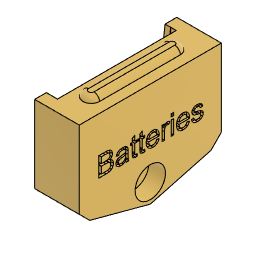
Battery_Cap (Autodesk Fusion 360 design; units mm, degrees)
Autodesk Fusion 360 part; units mm, degrees
(part 1 of 2)
sketch "Cap Face" plane through (-62, 0, 0) normal (-1, 0, 0) x (0, -1, 0)
  line L0 (0, -13.8691) -> (1.875, -15.7441)
  line L1 (1.875, -15.7441) -> (12.75, -18.6581)
  line L2 (12.75, -18.6581) -> (23.625, -15.7441)
  line L3 (23.625, -15.7441) -> (25.5, -13.8691)
  line L4 (0, 0) -> (25.5, 0)
  line L5 (25.5, 0) -> (25.5, -13.8691)
  line L6 (0, -13.8691) -> (0, 0)
  line L7 (0, -13.8691) -> (1.875, -15.7441)
  line L8 (1.875, -15.7441) -> (12.75, -18.6581)
  line L9 (12.75, -18.6581) -> (23.625, -15.7441)
  line L10 (23.625, -15.7441) -> (25.5, -13.8691)
  dimension "d72" = 13.8691
  dimension "d73" = 18.6581
  dimension "d74" = 25.5
  dimension "d75" = 10.875
  dimension "d76" = 10.875
  dimension "d77" = 1.875
  dimension "d78" = 1.875
  dimension "d79" = 1.875
  dimension "d80" = 1.875
  dimension "d81" = 2.9139
  dimension "d82" = 2.9139
  dimension "d83" = 150
  dimension "d84" = 150
  dimension "d85" = 135
  constraint coincident L4.start L6.end
  constraint horizontal L4
  constraint vertical L5
  constraint vertical L6
  constraint coincident L4.start L6
  constraint coincident L6.end L4
  constraint coincident L2 L1.end
  measures "d72" distance of L4.start L0.start
  measures "d73" vertical distance of L4.start L1.end
  measures "d74" distance of L4.start L4.end
  measures "d75" horizontal distance of L1.end L2.end
  measures "d76" horizontal distance of L0.end L1.end
  measures "d77" horizontal distance of L2.end L3.end
  measures "d78" horizontal distance of L0.end L0.start
  measures "d79" vertical distance of L2.end L3.end
  measures "d80" vertical distance of L0.end L0.start
  measures "d81" vertical distance of L1.end L2.end
  measures "d82" vertical distance of L0.end L1.end
  measures "d83" angle of L7 L8
  measures "d84" angle of L9 L10
  measures "d85" angle of L3 L5
extrude "Cap Extrusion" add sketch "Cap Face" along normal blind 8
sketch "Battery Label" plane through (-62, 0, 0) normal (1, 0, 0) x (0, 1, 0)
  line L0 (0, -13.8691) -> (0, 0)
  line L1 (0, 0) -> (-25.5, 0)
  line L2 (-25.5, 0) -> (-25.5, -13.8691)
  line L3 (-22, -10.5) -> (-3, -10.5) construction
  line L4 (-3, -10.5) -> (-3, -6.5) construction
  line L5 (-3, -6.5) -> (-22, -6.5) construction
  line L6 (-22, -6.5) -> (-22, -10.5) construction
  line L7 (-1.875, -15.7441) -> (0, -13.8691)
  line L8 (-25.5, -13.8691) -> (-23.625, -15.7441)
  line L9 (-23.625, -15.7441) -> (-12.75, -18.6581)
  line L10 (-12.75, -18.6581) -> (-1.875, -15.7441)
  dimension "d19" = 3.5
  dimension "d87" = 6.5
  dimension "d88" = 3.5
  dimension "d89" = 19
  dimension "d90" = 4
  text T0 "Batteries" font "Arial" height 3.5 align left top in box 19 x 4 at (-22, -10.5) x (1, 0) y (0, 1) spacing 1 kerned
  constraint parallel L1 L5
  measures "d87" distance of L1 L5
  measures "d88" distance of L2 L6
extrude "Label Cutout" cut sketch "Battery Label" against normal blind 0.5 text T0
sketch "Screw Hole" plane through (-62, 0, 0) normal (1, 0, 0) x (0, 1, 0)
  line L0 (0, -13.8691) -> (0, 0)
  line L1 (0, 0) -> (-25.5, 0)
  line L2 (-25.5, 0) -> (-25.5, -13.8691)
  spline S0 degree 3 poles (-20.1008, -9.9415) (-20.186, -9.9585) (-20.3723, -9.9958) (-20.5623, -9.9985) (-20.6654, -10) knots 0 0 0 0 0.026008 0.05687 0.05687 0.05687 0.05687
  line L3 (-20.6654, -10) -> (-22, -10)
  line L4 (-22, -10) -> (-22, -6.5)
  line L5 (-22, -6.5) -> (-20.6869, -6.5)
  spline S1 degree 3 poles (-20.6869, -6.5) (-20.5653, -6.5022) (-20.3453, -6.5062) (-20.1367, -6.5753) (-20.0435, -6.6062) knots 0 0 0 0 0.036237 0.065543 0.065543 0.065543 0.065543
  spline S2 degree 3 poles (-20.0435, -6.6062) (-19.9672, -6.6463) (-19.8153, -6.7259) (-19.7142, -6.8644) (-19.6639, -6.9333) knots 0 0 0 0 0.025471 0.050707 0.050707 0.050707 0.050707
  spline S3 degree 3 poles (-19.6639, -6.9333) (-19.6238, -7.0069) (-19.5453, -7.1513) (-19.5328, -7.3151) (-19.5266, -7.3953) knots 0 0 0 0 0.024827 0.048681 0.048681 0.048681 0.048681
  spline S4 degree 3 poles (-19.5266, -7.3953) (-19.5319, -7.4693) (-19.5425, -7.6188) (-19.6129, -7.7511) (-19.6484, -7.8179) knots 0 0 0 0 0.021997 0.044414 0.044414 0.044414 0.044414
  spline S5 degree 3 poles (-19.6484, -7.8179) (-19.6958, -7.8815) (-19.795, -8.0147) (-19.9402, -8.0956) (-20.016, -8.1378) knots 0 0 0 0 0.023539 0.049232 0.049232 0.049232 0.049232
  spline S6 degree 3 poles (-20.016, -8.1378) (-19.9177, -8.1726) (-19.7291, -8.2392) (-19.5929, -8.3854) (-19.5278, -8.4553) knots 0 0 0 0 0.030777 0.059013 0.059013 0.059013 0.059013
  spline S7 degree 3 poles (-19.5278, -8.4553) (-19.478, -8.5346) (-19.3762, -8.6966) (-19.3636, -8.8877) (-19.3571, -8.9853) knots 0 0 0 0 0.027618 0.056465 0.056465 0.056465 0.056465
  spline S8 degree 3 poles (-19.3571, -8.9853) (-19.3612, -9.0655) (-19.3694, -9.2239) (-19.4307, -9.3702) (-19.4609, -9.4425) knots 0 0 0 0 0.023867 0.0472 0.0472 0.0472 0.0472
  spline S9 degree 3 poles (-19.4609, -9.4425) (-19.4961, -9.5078) (-19.5627, -9.6315) (-19.6679, -9.7245) (-19.7176, -9.7684) knots 0 0 0 0 0.02202 0.041772 0.041772 0.041772 0.041772
  spline S10 degree 3 poles (-19.7176, -9.7684) (-19.7737, -9.8048) (-19.8926, -9.8817) (-20.0288, -9.9209) (-20.1008, -9.9415) knots 0 0 0 0 0.019941 0.042252 0.042252 0.042252 0.042252
  spline S11 degree 3 poles (-15.4524, -9.6013) (-15.4319, -9.6103) (-15.3853, -9.6308) (-15.3342, -9.6318) (-15.3056, -9.6323) knots 0 0 0 0 0.006657 0.015139 0.015139 0.015139 0.015139
  spline S12 degree 3 poles (-15.3056, -9.6323) (-15.2779, -9.6314) (-15.2148, -9.6291) (-15.1521, -9.6205) (-15.117, -9.6156) knots 0 0 0 0 0.008307 0.018945 0.018945 0.018945 0.018945
  line L6 (-15.117, -9.6156) -> (-15.0549, -9.9952)
  spline S13 degree 3 poles (-15.0549, -9.9952) (-15.112, -10.0064) (-15.2193, -10.0273) (-15.3285, -10.0315) (-15.3796, -10.0334) knots 0 0 0 0 0.017427 0.032736 0.032736 0.032736 0.032736
  spline S14 degree 3 poles (-15.3796, -10.0334) (-15.4499, -10.0321) (-15.5757, -10.0297) (-15.6914, -9.9809) (-15.7425, -9.9594) knots 0 0 0 0 0.020853 0.037334 0.037334 0.037334 0.037334
  spline S15 degree 3 poles (-15.7425, -9.9594) (-15.782, -9.9335) (-15.8584, -9.8834) (-15.9026, -9.8035) (-15.9239, -9.7648) knots 0 0 0 0 0.013927 0.026964 0.026964 0.026964 0.026964
  spline S16 degree 3 poles (-15.9239, -9.7648) (-15.939, -9.7027) (-15.9794, -9.5365) (-15.9776, -9.3649) (-15.9765, -9.2575) knots 0 0 0 0 0.019122 0.05117 0.05117 0.05117 0.05117
  line L7 (-15.9765, -9.2575) -> (-15.9765, -7.7988)
  line L8 (-15.9765, -7.7988) -> (-16.2916, -7.7988)
  line L9 (-16.2916, -7.7988) -> (-16.2916, -7.4645)
  line L10 (-16.2916, -7.4645) -> (-15.9765, -7.4645)
  line L11 (-15.9765, -7.4645) -> (-15.9765, -6.8366)
  line L12 (-15.9765, -6.8366) -> (-15.5491, -6.5788)
  line L13 (-15.5491, -6.5788) -> (-15.5491, -7.4645)
  line L14 (-15.5491, -7.4645) -> (-15.117, -7.4645)
  line L15 (-15.117, -7.4645) -> (-15.117, -7.7988)
  line L16 (-15.117, -7.7988) -> (-15.5491, -7.7988)
  line L17 (-15.5491, -7.7988) -> (-15.5491, -9.2814)
  spline S17 degree 3 poles (-15.5491, -9.2814) (-15.5497, -9.332) (-15.5507, -9.4118) (-15.5329, -9.4894) (-15.5264, -9.5177) knots 0 0 0 0 0.015111 0.023814 0.023814 0.023814 0.023814
  spline S18 degree 3 poles (-15.5264, -9.5177) (-15.5176, -9.5344) (-15.4996, -9.5682) (-15.4683, -9.5902) (-15.4524, -9.6013) knots 0 0 0 0 0.00558 0.011304 0.011304 0.011304 0.011304
  spline S19 degree 3 poles (-11.5477, -9.8424) (-11.6529, -9.905) (-11.876, -10.038) (-12.136, -10.0506) (-12.2735, -10.0573) knots 0 0 0 0 0.036142 0.076727 0.076727 0.076727 0.076727
  spline S20 degree 3 poles (-12.2735, -10.0573) (-12.4466, -10.0458) (-12.7775, -10.0239) (-13.0336, -9.8146) (-13.1557, -9.7147) knots 0 0 0 0 0.050598 0.096759 0.096759 0.096759 0.096759
  spline S21 degree 3 poles (-13.1557, -9.7147) (-13.2506, -9.5823) (-13.4557, -9.2963) (-13.4725, -8.9433) (-13.4816, -8.7538) knots 0 0 0 0 0.047865 0.103406 0.103406 0.103406 0.103406
  spline S22 degree 3 poles (-13.4816, -8.7538) (-13.4726, -8.5579) (-13.4561, -8.1943) (-13.2481, -7.8975) (-13.1521, -7.7606) knots 0 0 0 0 0.057415 0.106574 0.106574 0.106574 0.106574
  spline S23 degree 3 poles (-13.1521, -7.7606) (-13.0321, -7.6575) (-12.7864, -7.4464) (-12.463, -7.4205) (-12.2974, -7.4072) knots 0 0 0 0 0.046198 0.09464 0.09464 0.09464 0.09464
  spline S24 degree 3 poles (-12.2974, -7.4072) (-12.1368, -7.4204) (-11.8221, -7.4463) (-11.5834, -7.6525) (-11.4666, -7.7534) knots 0 0 0 0 0.047001 0.092108 0.092108 0.092108 0.092108
  spline S25 degree 3 poles (-14.094, -9.6013) (-14.0735, -9.6103) (-14.0268, -9.6308) (-13.9758, -9.6318) (-13.9471, -9.6323) knots 0 0 0 0 0.006657 0.015139 0.015139 0.015139 0.015139
  spline S26 degree 3 poles (-13.9471, -9.6323) (-13.9194, -9.6314) (-13.8563, -9.6291) (-13.7937, -9.6205) (-13.7585, -9.6156) knots 0 0 0 0 0.008307 0.018945 0.018945 0.018945 0.018945
  line L18 (-13.7585, -9.6156) -> (-13.6965, -9.9952)
  spline S27 degree 3 poles (-13.6965, -9.9952) (-13.7536, -10.0064) (-13.8609, -10.0273) (-13.9701, -10.0315) (-14.0211, -10.0334) knots 0 0 0 0 0.017427 0.032736 0.032736 0.032736 0.032736
  spline S28 degree 3 poles (-14.0211, -10.0334) (-14.0914, -10.0321) (-14.2173, -10.0297) (-14.333, -9.9809) (-14.384, -9.9594) knots 0 0 0 0 0.020853 0.037334 0.037334 0.037334 0.037334
  spline S29 degree 3 poles (-14.384, -9.9594) (-14.4235, -9.9335) (-14.4999, -9.8834) (-14.5441, -9.8035) (-14.5655, -9.7648) knots 0 0 0 0 0.013927 0.026964 0.026964 0.026964 0.026964
  spline S30 degree 3 poles (-14.5655, -9.7648) (-14.5806, -9.7027) (-14.621, -9.5365) (-14.6192, -9.3649) (-14.618, -9.2575) knots 0 0 0 0 0.019122 0.05117 0.05117 0.05117 0.05117
  line L19 (-14.618, -9.2575) -> (-14.618, -7.7988)
  line L20 (-14.618, -7.7988) -> (-14.9332, -7.7988)
  line L21 (-14.9332, -7.7988) -> (-14.9332, -7.4645)
  line L22 (-14.9332, -7.4645) -> (-14.618, -7.4645)
  line L23 (-14.618, -7.4645) -> (-14.618, -6.8366)
  line L24 (-14.618, -6.8366) -> (-14.1907, -6.5788)
  line L25 (-14.1907, -6.5788) -> (-14.1907, -7.4645)
  line L26 (-14.1907, -7.4645) -> (-13.7585, -7.4645)
  line L27 (-13.7585, -7.4645) -> (-13.7585, -7.7988)
  line L28 (-13.7585, -7.7988) -> (-14.1907, -7.7988)
  line L29 (-14.1907, -7.7988) -> (-14.1907, -9.2814)
  spline S31 degree 3 poles (-14.1907, -9.2814) (-14.1913, -9.332) (-14.1923, -9.4118) (-14.1745, -9.4894) (-14.168, -9.5177) knots 0 0 0 0 0.015111 0.023814 0.023814 0.023814 0.023814
  spline S32 degree 3 poles (-14.168, -9.5177) (-14.1591, -9.5344) (-14.1412, -9.5682) (-14.1098, -9.5902) (-14.094, -9.6013) knots 0 0 0 0 0.00558 0.011304 0.011304 0.011304 0.011304
  line L30 (-16.5853, -10) -> (-17.0341, -10)
  spline S33 degree 3 poles (-17.0341, -10) (-17.0545, -9.9522) (-17.0974, -9.852) (-17.1123, -9.7439) (-17.1201, -9.6872) knots 0 0 0 0 0.015508 0.032565 0.032565 0.032565 0.032565
  spline S34 degree 3 poles (-17.1201, -9.6872) (-17.1958, -9.7487) (-17.3372, -9.8634) (-17.5028, -9.9388) (-17.5796, -9.9737) knots 0 0 0 0 0.029128 0.054352 0.054352 0.054352 0.054352
  spline S35 degree 3 poles (-17.5796, -9.9737) (-17.6553, -9.9981) (-17.8094, -10.0477) (-17.9712, -10.0541) (-18.0535, -10.0573) knots 0 0 0 0 0.023732 0.048322 0.048322 0.048322 0.048322
  spline S36 degree 3 poles (-18.0535, -10.0573) (-18.1807, -10.0522) (-18.4145, -10.0429) (-18.6077, -9.9126) (-18.6958, -9.8532) knots 0 0 0 0 0.037297 0.068576 0.068576 0.068576 0.068576
  spline S37 degree 3 poles (-18.6958, -9.8532) (-18.7612, -9.7797) (-18.8939, -9.6309) (-18.9113, -9.4322) (-18.9202, -9.3315) knots 0 0 0 0 0.028701 0.058158 0.058158 0.058158 0.058158
  spline S38 degree 3 poles (-18.9202, -9.3315) (-18.9169, -9.2712) (-18.9104, -9.1523) (-18.8602, -9.0444) (-18.8354, -8.9913) knots 0 0 0 0 0.017942 0.035349 0.035349 0.035349 0.035349
  spline S39 degree 3 poles (-18.8354, -8.9913) (-18.8054, -8.9428) (-18.7461, -8.8471) (-18.6572, -8.7782) (-18.6134, -8.7442) knots 0 0 0 0 0.016982 0.033459 0.033459 0.033459 0.033459
  spline S40 degree 3 poles (-18.6134, -8.7442) (-18.5657, -8.7149) (-18.4685, -8.6552) (-18.3596, -8.6209) (-18.3042, -8.6033) knots 0 0 0 0 0.016728 0.034089 0.034089 0.034089 0.034089
  spline S41 degree 3 poles (-18.3042, -8.6033) (-18.2514, -8.5917) (-18.1252, -8.5639) (-17.9969, -8.5481) (-17.9222, -8.5389) knots 0 0 0 0 0.016212 0.038758 0.038758 0.038758 0.038758
  spline S42 degree 3 poles (-17.9222, -8.5389) (-17.7708, -8.5205) (-17.5117, -8.4892) (-17.2603, -8.4197) (-17.1559, -8.3909) knots 0 0 0 0 0.045692 0.078147 0.078147 0.078147 0.078147
  spline S43 degree 3 poles (-17.1559, -8.3909) (-17.1552, -8.3668) (-17.1541, -8.3294) (-17.1537, -8.292) (-17.1535, -8.2786) knots 0 0 0 0 0.007224 0.011224 0.011224 0.011224 0.011224
  spline S44 degree 3 poles (-17.1535, -8.2786) (-17.1552, -8.201) (-17.1582, -8.0641) (-17.2399, -7.9556) (-17.2752, -7.9086) knots 0 0 0 0 0.022588 0.039829 0.039829 0.039829 0.039829
  spline S45 degree 3 poles (-17.2752, -7.9086) (-17.3416, -7.8662) (-17.49, -7.7715) (-17.6669, -7.766) (-17.7647, -7.763) knots 0 0 0 0 0.023204 0.051906 0.051906 0.051906 0.051906
  spline S46 degree 3 poles (-17.7647, -7.763) (-17.8544, -7.7644) (-18.0122, -7.7668) (-18.152, -7.8384) (-18.2123, -7.8692) knots 0 0 0 0 0.026485 0.046548 0.046548 0.046548 0.046548
  spline S47 degree 3 poles (-18.2123, -7.8692) (-18.2583, -7.9158) (-18.3627, -8.0214) (-18.4033, -8.165) (-18.426, -8.2452) knots 0 0 0 0 0.019347 0.043872 0.043872 0.043872 0.043872
  line L31 (-18.426, -8.2452) -> (-18.8462, -8.1879)
  spline S48 degree 3 poles (-18.8462, -8.1879) (-18.8257, -8.1045) (-18.7873, -7.9485) (-18.6988, -7.8146) (-18.6576, -7.7522) knots 0 0 0 0 0.025533 0.047792 0.047792 0.047792 0.047792
  spline S49 degree 3 poles (-18.6576, -7.7522) (-18.6067, -7.6993) (-18.4988, -7.587) (-18.3544, -7.528) (-18.278, -7.4968) knots 0 0 0 0 0.021757 0.046207 0.046207 0.046207 0.046207
  spline S50 degree 3 poles (-18.278, -7.4968) (-18.1892, -7.4707) (-18.0015, -7.4155) (-17.8058, -7.4101) (-17.7026, -7.4072) knots 0 0 0 0 0.027628 0.058447 0.058447 0.058447 0.058447
  spline S51 degree 3 poles (-17.7026, -7.4072) (-17.6038, -7.4089) (-17.4245, -7.4119) (-17.2523, -7.4614) (-17.175, -7.4836) knots 0 0 0 0 0.029487 0.053518 0.053518 0.053518 0.053518
  spline S52 degree 3 poles (-17.175, -7.4836) (-17.1137, -7.5085) (-17.0019, -7.554) (-16.9156, -7.6379) (-16.8765, -7.6758) knots 0 0 0 0 0.019606 0.035791 0.035791 0.035791 0.035791
  spline S53 degree 3 poles (-16.8765, -7.6758) (-16.8468, -7.7183) (-16.7844, -7.8074) (-16.7571, -7.913) (-16.7428, -7.9683) knots 0 0 0 0 0.015412 0.03239 0.03239 0.03239 0.03239
  spline S54 degree 3 poles (-16.7428, -7.9683) (-16.7366, -8.0196) (-16.7207, -8.1511) (-16.7211, -8.2837) (-16.7214, -8.3646) knots 0 0 0 0 0.015483 0.039722 0.039722 0.039722 0.039722
  line L32 (-16.7214, -8.3646) -> (-16.7214, -8.9376)
  spline S55 degree 3 poles (-16.7214, -8.9376) (-16.7223, -9.1008) (-16.7239, -9.3539) (-16.7018, -9.606) (-16.6939, -9.6956) knots 0 0 0 0 0.048918 0.075885 0.075885 0.075885 0.075885
  spline S56 degree 3 poles (-16.6939, -9.6956) (-16.6824, -9.7482) (-16.6592, -9.8543) (-16.61, -9.9511) (-16.5853, -10) knots 0 0 0 0 0.016077 0.032437 0.032437 0.032437 0.032437
  circle A0 centre (-12.75, -15.2374) radius 1.4264
  spline S57 degree 3 poles (-12.2711, -9.704) (-12.1963, -9.6995) (-12.0515, -9.691) (-11.9275, -9.616) (-11.8677, -9.5798) knots 0 0 0 0 0.022124 0.042784 0.042784 0.042784 0.042784
  spline S58 degree 3 poles (-11.8677, -9.5798) (-11.8137, -9.5289) (-11.6955, -9.4173) (-11.6353, -9.2658) (-11.6027, -9.1835) knots 0 0 0 0 0.022003 0.048189 0.048189 0.048189 0.048189
  line L33 (-11.6027, -9.1835) -> (-11.1586, -9.2384)
  spline S59 degree 3 poles (-11.1586, -9.2384) (-11.1994, -9.3596) (-11.2783, -9.594) (-11.46, -9.7615) (-11.5477, -9.8424) knots 0 0 0 0 0.037666 0.07289 0.07289 0.07289 0.07289
  spline S60 degree 3 poles (-11.4666, -7.7534) (-11.3727, -7.8877) (-11.1691, -8.1789) (-11.153, -8.5354) (-11.1443, -8.7275) knots 0 0 0 0 0.048166 0.104492 0.104492 0.104492 0.104492
  spline S61 degree 3 poles (-11.1443, -8.7275) (-11.1444, -8.7434) (-11.1448, -8.7816) (-11.146, -8.8198) (-11.1467, -8.8421) knots 0 0 0 0 0.004775 0.011463 0.011463 0.011463 0.011463
  line L34 (-11.1467, -8.8421) -> (-13.0375, -8.8421)
  spline S62 degree 3 poles (-13.0375, -8.8421) (-13.0251, -8.9694) (-13.0022, -9.2043) (-12.8643, -9.3947) (-12.8012, -9.4819) knots 0 0 0 0 0.037564 0.069307 0.069307 0.069307 0.069307
  spline S63 degree 3 poles (-12.8012, -9.4819) (-12.7255, -9.5467) (-12.5727, -9.6774) (-12.3723, -9.6951) (-12.2711, -9.704) knots 0 0 0 0 0.029108 0.058759 0.058759 0.058759 0.058759
  line L35 (-10.1941, -8.6726) -> (-10.1941, -10)
  line L36 (-10.1941, -10) -> (-10.6238, -10)
  line L37 (-10.6238, -10) -> (-10.6238, -7.4645)
  line L38 (-10.6238, -7.4645) -> (-10.237, -7.4645)
  line L39 (-10.237, -7.4645) -> (-10.237, -7.8489)
  spline S64 degree 3 poles (-10.237, -7.8489) (-10.194, -7.7708) (-10.1207, -7.638) (-10.0095, -7.5354) (-9.9637, -7.4932) knots 0 0 0 0 0.026526 0.045117 0.045117 0.045117 0.045117
  spline S65 degree 3 poles (-9.9637, -7.4932) (-9.9209, -7.4681) (-9.8356, -7.4181) (-9.7371, -7.4109) (-9.6879, -7.4072) knots 0 0 0 0 0.014655 0.029228 0.029228 0.029228 0.029228
  spline S66 degree 3 poles (-9.6879, -7.4072) (-9.6135, -7.4141) (-9.4566, -7.4286) (-9.3187, -7.5053) (-9.2462, -7.5457) knots 0 0 0 0 0.022177 0.046743 0.046743 0.046743 0.046743
  line L40 (-9.2462, -7.5457) -> (-9.3943, -7.9444)
  spline S67 degree 3 poles (-9.3943, -7.9444) (-9.4457, -7.9173) (-9.5446, -7.865) (-9.6559, -7.8558) (-9.7094, -7.8513) knots 0 0 0 0 0.017235 0.033164 0.033164 0.033164 0.033164
  spline S68 degree 3 poles (-9.7094, -7.8513) (-9.7552, -7.8548) (-9.8466, -7.8619) (-9.9239, -7.9113) (-9.9625, -7.9361) knots 0 0 0 0 0.013537 0.027061 0.027061 0.027061 0.027061
  spline S69 degree 3 poles (-9.9625, -7.9361) (-9.9974, -7.9678) (-10.0695, -8.0332) (-10.1045, -8.1243) (-10.1224, -8.1712) knots 0 0 0 0 0.013953 0.028797 0.028797 0.028797 0.028797
  spline S70 degree 3 poles (-10.1224, -8.1712) (-10.1433, -8.2508) (-10.1865, -8.4151) (-10.1915, -8.5849) (-10.1941, -8.6726) knots 0 0 0 0 0.024588 0.050792 0.050792 0.050792 0.050792
  line L41 (-8.5587, -7.4645) -> (-8.5587, -10)
  line L42 (-8.5587, -10) -> (-8.9884, -10)
  line L43 (-8.9884, -10) -> (-8.9884, -7.4645)
  line L44 (-8.9884, -7.4645) -> (-8.5587, -7.4645)
  spline S71 degree 3 poles (-6.8373, -9.704) (-6.7624, -9.6995) (-6.6176, -9.691) (-6.4937, -9.616) (-6.4338, -9.5798) knots 0 0 0 0 0.022124 0.042784 0.042784 0.042784 0.042784
  spline S72 degree 3 poles (-6.4338, -9.5798) (-6.3799, -9.5289) (-6.2617, -9.4173) (-6.2015, -9.2658) (-6.1688, -9.1835) knots 0 0 0 0 0.022003 0.048189 0.048189 0.048189 0.048189
  line L45 (-6.1688, -9.1835) -> (-5.7248, -9.2384)
  spline S73 degree 3 poles (-5.7248, -9.2384) (-5.7656, -9.3596) (-5.8445, -9.594) (-6.0261, -9.7615) (-6.1139, -9.8424) knots 0 0 0 0 0.037666 0.07289 0.07289 0.07289 0.07289
  spline S74 degree 3 poles (-6.1139, -9.8424) (-6.219, -9.905) (-6.4422, -10.038) (-6.7022, -10.0506) (-6.8397, -10.0573) knots 0 0 0 0 0.036142 0.076727 0.076727 0.076727 0.076727
  spline S75 degree 3 poles (-6.8397, -10.0573) (-7.0128, -10.0458) (-7.3437, -10.0239) (-7.5997, -9.8146) (-7.7219, -9.7147) knots 0 0 0 0 0.050598 0.096759 0.096759 0.096759 0.096759
  spline S76 degree 3 poles (-7.7219, -9.7147) (-7.8168, -9.5823) (-8.0218, -9.2963) (-8.0387, -8.9433) (-8.0478, -8.7538) knots 0 0 0 0 0.047864 0.103406 0.103406 0.103406 0.103406
  spline S77 degree 3 poles (-8.0478, -8.7538) (-8.0388, -8.5579) (-8.0222, -8.1943) (-7.8142, -7.8975) (-7.7183, -7.7606) knots 0 0 0 0 0.057415 0.106574 0.106574 0.106574 0.106574
  spline S78 degree 3 poles (-7.7183, -7.7606) (-7.5983, -7.6575) (-7.3526, -7.4464) (-7.0291, -7.4205) (-6.8636, -7.4072) knots 0 0 0 0 0.046198 0.09464 0.09464 0.09464 0.09464
  spline S79 degree 3 poles (-6.8636, -7.4072) (-6.703, -7.4204) (-6.3883, -7.4463) (-6.1496, -7.6525) (-6.0327, -7.7534) knots 0 0 0 0 0.047001 0.092108 0.092108 0.092108 0.092108
  spline S80 degree 3 poles (-6.0327, -7.7534) (-5.9389, -7.8877) (-5.7353, -8.1789) (-5.7191, -8.5354) (-5.7104, -8.7275) knots 0 0 0 0 0.048166 0.104492 0.104492 0.104492 0.104492
  spline S81 degree 3 poles (-5.7104, -8.7275) (-5.7106, -8.7434) (-5.711, -8.7816) (-5.7121, -8.8198) (-5.7128, -8.8421) knots 0 0 0 0 0.004775 0.011463 0.011463 0.011463 0.011463
  line L46 (-5.7128, -8.8421) -> (-7.6037, -8.8421)
  spline S82 degree 3 poles (-7.6037, -8.8421) (-7.5913, -8.9694) (-7.5684, -9.2043) (-7.4305, -9.3947) (-7.3673, -9.4819) knots 0 0 0 0 0.037564 0.069307 0.069307 0.069307 0.069307
  spline S83 degree 3 poles (-7.3673, -9.4819) (-7.2916, -9.5467) (-7.1389, -9.6774) (-6.9384, -9.6951) (-6.8373, -9.704) knots 0 0 0 0 0.029108 0.058759 0.058759 0.058759 0.058759
  line L47 (-8.5587, -6.5) -> (-8.5587, -6.9942)
  line L48 (-8.5587, -6.9942) -> (-8.9884, -6.9942)
  line L49 (-8.9884, -6.9942) -> (-8.9884, -6.5)
  line L50 (-8.9884, -6.5) -> (-8.5587, -6.5)
  spline S84 degree 3 poles (-4.2732, -10.0573) (-4.4221, -10.0531) (-4.691, -10.0455) (-4.9229, -9.9117) (-5.0264, -9.852) knots 0 0 0 0 0.043843 0.07916 0.07916 0.07916 0.07916
  spline S85 degree 3 poles (-5.0264, -9.852) (-5.1055, -9.7717) (-5.2737, -9.6011) (-5.3282, -9.3671) (-5.3571, -9.2432) knots 0 0 0 0 0.033163 0.070487 0.070487 0.070487 0.070487
  line L51 (-5.3571, -9.2432) -> (-4.9321, -9.1763)
  spline S86 degree 3 poles (-4.9321, -9.1763) (-4.9164, -9.2551) (-4.8867, -9.4048) (-4.7822, -9.5155) (-4.7328, -9.5679) knots 0 0 0 0 0.023556 0.044735 0.044735 0.044735 0.044735
  spline S87 degree 3 poles (-4.7328, -9.5679) (-4.6692, -9.6075) (-4.5298, -9.6943) (-4.3651, -9.7006) (-4.2756, -9.704) knots 0 0 0 0 0.022104 0.048438 0.048438 0.048438 0.048438
  spline S88 degree 3 poles (-4.2756, -9.704) (-4.1872, -9.7019) (-4.0299, -9.6983) (-3.8953, -9.6184) (-3.8363, -9.5834) knots 0 0 0 0 0.02596 0.046233 0.046233 0.046233 0.046233
  spline S89 degree 3 poles (-3.8363, -9.5834) (-3.7945, -9.5427) (-3.7143, -9.4644) (-3.6999, -9.3536) (-3.693, -9.3005) knots 0 0 0 0 0.016943 0.032549 0.032549 0.032549 0.032549
  spline S90 degree 3 poles (-3.693, -9.3005) (-3.6986, -9.2544) (-3.7098, -9.161) (-3.7827, -9.1014) (-3.8196, -9.0713) knots 0 0 0 0 0.013391 0.02711 0.02711 0.02711 0.02711
  spline S91 degree 3 poles (-3.8196, -9.0713) (-3.8705, -9.0484) (-4.0117, -8.985) (-4.1625, -8.9488) (-4.2589, -8.9256) knots 0 0 0 0 0.016717 0.046363 0.046363 0.046363 0.046363
  spline S92 degree 3 poles (-4.2589, -8.9256) (-4.3934, -8.892) (-4.6161, -8.8362) (-4.8296, -8.7523) (-4.9142, -8.7191) knots 0 0 0 0 0.041539 0.068773 0.068773 0.068773 0.068773
  spline S93 degree 3 poles (-4.9142, -8.7191) (-4.9709, -8.6881) (-5.081, -8.6279) (-5.1552, -8.527) (-5.1912, -8.478) knots 0 0 0 0 0.019122 0.037119 0.037119 0.037119 0.037119
  spline S94 degree 3 poles (-5.1912, -8.478) (-5.2187, -8.4251) (-5.2741, -8.3184) (-5.2817, -8.1983) (-5.2855, -8.1378) knots 0 0 0 0 0.017681 0.035653 0.035653 0.035653 0.035653
  spline S95 degree 3 poles (-5.2855, -8.1378) (-5.2824, -8.0825) (-5.2762, -7.973) (-5.2305, -7.8733) (-5.2079, -7.8238) knots 0 0 0 0 0.016439 0.032594 0.032594 0.032594 0.032594
  spline S96 degree 3 poles (-5.2079, -7.8238) (-5.1797, -7.7777) (-5.1232, -7.6854) (-5.0388, -7.6178) (-4.9966, -7.5839) knots 0 0 0 0 0.016085 0.032187 0.032187 0.032187 0.032187
  spline S97 degree 3 poles (-4.9966, -7.5839) (-4.9578, -7.5595) (-4.8723, -7.5057) (-4.7759, -7.4752) (-4.7232, -7.4586) knots 0 0 0 0 0.013677 0.030182 0.030182 0.030182 0.030182
  spline S98 degree 3 poles (-4.7232, -7.4586) (-4.6637, -7.4436) (-4.5419, -7.4129) (-4.4163, -7.4092) (-4.352, -7.4072) knots 0 0 0 0 0.018344 0.037576 0.037576 0.037576 0.037576
  spline S99 degree 3 poles (-4.352, -7.4072) (-4.2578, -7.41) (-4.0792, -7.4152) (-3.9086, -7.4681) (-3.8279, -7.4932) knots 0 0 0 0 0.028105 0.053325 0.053325 0.053325 0.053325
  spline S100 degree 3 poles (-3.8279, -7.4932) (-3.7593, -7.5223) (-3.6315, -7.5764) (-3.5381, -7.6787) (-3.4949, -7.726) knots 0 0 0 0 0.022063 0.041059 0.041059 0.041059 0.041059
  spline S101 degree 3 poles (-3.4949, -7.726) (-3.4614, -7.7819) (-3.3886, -7.9037) (-3.3615, -8.0432) (-3.3469, -8.1187) knots 0 0 0 0 0.01941 0.042254 0.042254 0.042254 0.042254
  line L52 (-3.3469, -8.1187) -> (-3.7671, -8.176)
  spline S102 degree 3 poles (-3.7671, -8.176) (-3.7803, -8.115) (-3.8061, -7.9968) (-3.8916, -7.9116) (-3.933, -7.8704) knots 0 0 0 0 0.0183 0.035437 0.035437 0.035437 0.035437
  spline S103 degree 3 poles (-3.933, -7.8704) (-3.9868, -7.8384) (-4.1059, -7.7678) (-4.2448, -7.7631) (-4.3209, -7.7606) knots 0 0 0 0 0.018498 0.0409 0.0409 0.0409 0.0409
  spline S104 degree 3 poles (-4.3209, -7.7606) (-4.4074, -7.7613) (-4.5564, -7.7625) (-4.6882, -7.8301) (-4.7435, -7.8585) knots 0 0 0 0 0.025484 0.043902 0.043902 0.043902 0.043902
  spline S105 degree 3 poles (-4.7435, -7.8585) (-4.7804, -7.8911) (-4.8501, -7.9528) (-4.8637, -8.0444) (-4.8701, -8.0877) knots 0 0 0 0 0.014246 0.026941 0.026941 0.026941 0.026941
  spline S106 degree 3 poles (-4.8701, -8.0877) (-4.8678, -8.1149) (-4.8633, -8.1695) (-4.8329, -8.2151) (-4.8175, -8.2381) knots 0 0 0 0 0.008046 0.016168 0.016168 0.016168 0.016168
  spline S107 degree 3 poles (-4.8175, -8.2381) (-4.7961, -8.2607) (-4.7493, -8.3102) (-4.6868, -8.3377) (-4.6528, -8.3527) knots 0 0 0 0 0.009247 0.020247 0.020247 0.020247 0.020247
  spline S108 degree 3 poles (-4.6528, -8.3527) (-4.6105, -8.366) (-4.4848, -8.4056) (-4.3576, -8.4398) (-4.2732, -8.4625) knots 0 0 0 0 0.01331 0.039521 0.039521 0.039521 0.039521
  spline S109 degree 3 poles (-4.2732, -8.4625) (-4.1434, -8.497) (-3.9283, -8.5541) (-3.7197, -8.6312) (-3.6369, -8.6618) knots 0 0 0 0 0.040259 0.066707 0.066707 0.066707 0.066707
  spline S110 degree 3 poles (-3.6369, -8.6618) (-3.5805, -8.6901) (-3.4701, -8.7452) (-3.3921, -8.8408) (-3.354, -8.8874) knots 0 0 0 0 0.018692 0.036554 0.036554 0.036554 0.036554
  spline S111 degree 3 poles (-3.354, -8.8874) (-3.3241, -8.9415) (-3.2609, -9.0557) (-3.2547, -9.1864) (-3.2514, -9.2551) knots 0 0 0 0 0.018292 0.038629 0.038629 0.038629 0.038629
  spline S112 degree 3 poles (-3.2514, -9.2551) (-3.2569, -9.3262) (-3.2681, -9.4704) (-3.3402, -9.596) (-3.3767, -9.6598) knots 0 0 0 0 0.021094 0.042838 0.042838 0.042838 0.042838
  spline S113 degree 3 poles (-3.3767, -9.6598) (-3.4244, -9.72) (-3.523, -9.8446) (-3.665, -9.9164) (-3.7384, -9.9534) knots 0 0 0 0 0.022753 0.047089 0.047089 0.047089 0.047089
  spline S114 degree 3 poles (-3.7384, -9.9534) (-3.8215, -9.9837) (-3.9942, -10.0466) (-4.1779, -10.0537) (-4.2732, -10.0573) knots 0 0 0 0 0.026364 0.054775 0.054775 0.054775 0.054775
  line L53 (-1.875, -15.7441) -> (0, -13.8691)
  line L54 (-25.5, -13.8691) -> (-23.625, -15.7441)
  line L55 (-23.625, -15.7441) -> (-12.75, -18.6581)
  line L56 (-12.75, -18.6581) -> (-1.875, -15.7441)
  point P0 (-12.75, -13.811)
  dimension "d92" = 12.75
  dimension "d93" = 2.8528
  dimension "d94" = 13.811
  constraint coincident A0 P0
  constraint collinear A0.centre L55.end P0
  measures "d92" distance of L2 A0.centre
  measures "d93" diameter of A0
  measures "d94" distance of L1 P0
extrude "Screw Hole Cutout" cut sketch "Screw Hole" against normal blind 9 contours A0
sketch "Countersink" plane through (-62, 0, 0) normal (1, 0, 0) x (0, 1, 0)
  line L0 (0, -13.8691) -> (0, 0)
  line L1 (0, 0) -> (-25.5, 0)
  line L2 (-25.5, 0) -> (-25.5, -13.8691)
  spline S0 degree 3 poles (-20.1008, -9.9415) (-20.186, -9.9585) (-20.3723, -9.9958) (-20.5623, -9.9985) (-20.6654, -10) knots 0 0 0 0 0.026008 0.05687 0.05687 0.05687 0.05687
  line L3 (-20.6654, -10) -> (-22, -10)
  line L4 (-22, -10) -> (-22, -6.5)
  line L5 (-22, -6.5) -> (-20.6869, -6.5)
  spline S1 degree 3 poles (-20.6869, -6.5) (-20.5653, -6.5022) (-20.3453, -6.5062) (-20.1367, -6.5753) (-20.0435, -6.6062) knots 0 0 0 0 0.036237 0.065543 0.065543 0.065543 0.065543
  spline S2 degree 3 poles (-20.0435, -6.6062) (-19.9672, -6.6463) (-19.8153, -6.7259) (-19.7142, -6.8644) (-19.6639, -6.9333) knots 0 0 0 0 0.025471 0.050707 0.050707 0.050707 0.050707
  spline S3 degree 3 poles (-19.6639, -6.9333) (-19.6238, -7.0069) (-19.5453, -7.1513) (-19.5328, -7.3151) (-19.5266, -7.3953) knots 0 0 0 0 0.024827 0.048681 0.048681 0.048681 0.048681
  spline S4 degree 3 poles (-19.5266, -7.3953) (-19.5319, -7.4693) (-19.5425, -7.6188) (-19.6129, -7.7511) (-19.6484, -7.8179) knots 0 0 0 0 0.021997 0.044414 0.044414 0.044414 0.044414
  spline S5 degree 3 poles (-19.6484, -7.8179) (-19.6958, -7.8815) (-19.795, -8.0147) (-19.9402, -8.0956) (-20.016, -8.1378) knots 0 0 0 0 0.023539 0.049232 0.049232 0.049232 0.049232
  spline S6 degree 3 poles (-20.016, -8.1378) (-19.9177, -8.1726) (-19.7291, -8.2392) (-19.5929, -8.3854) (-19.5278, -8.4553) knots 0 0 0 0 0.030777 0.059013 0.059013 0.059013 0.059013
  spline S7 degree 3 poles (-19.5278, -8.4553) (-19.478, -8.5346) (-19.3762, -8.6966) (-19.3636, -8.8877) (-19.3571, -8.9853) knots 0 0 0 0 0.027618 0.056465 0.056465 0.056465 0.056465
  spline S8 degree 3 poles (-19.3571, -8.9853) (-19.3612, -9.0655) (-19.3694, -9.2239) (-19.4307, -9.3702) (-19.4609, -9.4425) knots 0 0 0 0 0.023867 0.0472 0.0472 0.0472 0.0472
  spline S9 degree 3 poles (-19.4609, -9.4425) (-19.4961, -9.5078) (-19.5627, -9.6315) (-19.6679, -9.7245) (-19.7176, -9.7684) knots 0 0 0 0 0.02202 0.041772 0.041772 0.041772 0.041772
  spline S10 degree 3 poles (-19.7176, -9.7684) (-19.7737, -9.8048) (-19.8926, -9.8817) (-20.0288, -9.9209) (-20.1008, -9.9415) knots 0 0 0 0 0.019941 0.042252 0.042252 0.042252 0.042252
  spline S11 degree 3 poles (-15.4524, -9.6013) (-15.4319, -9.6103) (-15.3853, -9.6308) (-15.3342, -9.6318) (-15.3056, -9.6323) knots 0 0 0 0 0.006657 0.015139 0.015139 0.015139 0.015139
  spline S12 degree 3 poles (-15.3056, -9.6323) (-15.2779, -9.6314) (-15.2148, -9.6291) (-15.1521, -9.6205) (-15.117, -9.6156) knots 0 0 0 0 0.008307 0.018945 0.018945 0.018945 0.018945
  line L6 (-15.117, -9.6156) -> (-15.0549, -9.9952)
  spline S13 degree 3 poles (-15.0549, -9.9952) (-15.112, -10.0064) (-15.2193, -10.0273) (-15.3285, -10.0315) (-15.3796, -10.0334) knots 0 0 0 0 0.017427 0.032736 0.032736 0.032736 0.032736
  spline S14 degree 3 poles (-15.3796, -10.0334) (-15.4499, -10.0321) (-15.5757, -10.0297) (-15.6914, -9.9809) (-15.7425, -9.9594) knots 0 0 0 0 0.020853 0.037334 0.037334 0.037334 0.037334
  spline S15 degree 3 poles (-15.7425, -9.9594) (-15.782, -9.9335) (-15.8584, -9.8834) (-15.9026, -9.8035) (-15.9239, -9.7648) knots 0 0 0 0 0.013927 0.026964 0.026964 0.026964 0.026964
  spline S16 degree 3 poles (-15.9239, -9.7648) (-15.939, -9.7027) (-15.9794, -9.5365) (-15.9776, -9.3649) (-15.9765, -9.2575) knots 0 0 0 0 0.019122 0.05117 0.05117 0.05117 0.05117
  line L7 (-15.9765, -9.2575) -> (-15.9765, -7.7988)
  line L8 (-15.9765, -7.7988) -> (-16.2916, -7.7988)
  line L9 (-16.2916, -7.7988) -> (-16.2916, -7.4645)
  line L10 (-16.2916, -7.4645) -> (-15.9765, -7.4645)
  line L11 (-15.9765, -7.4645) -> (-15.9765, -6.8366)
  line L12 (-15.9765, -6.8366) -> (-15.5491, -6.5788)
  line L13 (-15.5491, -6.5788) -> (-15.5491, -7.4645)
  line L14 (-15.5491, -7.4645) -> (-15.117, -7.4645)
  line L15 (-15.117, -7.4645) -> (-15.117, -7.7988)
  line L16 (-15.117, -7.7988) -> (-15.5491, -7.7988)
  line L17 (-15.5491, -7.7988) -> (-15.5491, -9.2814)
  spline S17 degree 3 poles (-15.5491, -9.2814) (-15.5497, -9.332) (-15.5507, -9.4118) (-15.5329, -9.4894) (-15.5264, -9.5177) knots 0 0 0 0 0.015111 0.023814 0.023814 0.023814 0.023814
  spline S18 degree 3 poles (-15.5264, -9.5177) (-15.5176, -9.5344) (-15.4996, -9.5682) (-15.4683, -9.5902) (-15.4524, -9.6013) knots 0 0 0 0 0.00558 0.011304 0.011304 0.011304 0.011304
  spline S19 degree 3 poles (-11.5477, -9.8424) (-11.6529, -9.905) (-11.876, -10.038) (-12.136, -10.0506) (-12.2735, -10.0573) knots 0 0 0 0 0.036142 0.076727 0.076727 0.076727 0.076727
  spline S20 degree 3 poles (-12.2735, -10.0573) (-12.4466, -10.0458) (-12.7775, -10.0239) (-13.0336, -9.8146) (-13.1557, -9.7147) knots 0 0 0 0 0.050598 0.096759 0.096759 0.096759 0.096759
  spline S21 degree 3 poles (-13.1557, -9.7147) (-13.2506, -9.5823) (-13.4557, -9.2963) (-13.4725, -8.9433) (-13.4816, -8.7538) knots 0 0 0 0 0.047865 0.103406 0.103406 0.103406 0.103406
  spline S22 degree 3 poles (-13.4816, -8.7538) (-13.4726, -8.5579) (-13.4561, -8.1943) (-13.2481, -7.8975) (-13.1521, -7.7606) knots 0 0 0 0 0.057415 0.106574 0.106574 0.106574 0.106574
  spline S23 degree 3 poles (-13.1521, -7.7606) (-13.0321, -7.6575) (-12.7864, -7.4464) (-12.463, -7.4205) (-12.2974, -7.4072) knots 0 0 0 0 0.046198 0.09464 0.09464 0.09464 0.09464
  spline S24 degree 3 poles (-12.2974, -7.4072) (-12.1368, -7.4204) (-11.8221, -7.4463) (-11.5834, -7.6525) (-11.4666, -7.7534) knots 0 0 0 0 0.047001 0.092108 0.092108 0.092108 0.092108
  spline S25 degree 3 poles (-14.094, -9.6013) (-14.0735, -9.6103) (-14.0268, -9.6308) (-13.9758, -9.6318) (-13.9471, -9.6323) knots 0 0 0 0 0.006657 0.015139 0.015139 0.015139 0.015139
  spline S26 degree 3 poles (-13.9471, -9.6323) (-13.9194, -9.6314) (-13.8563, -9.6291) (-13.7937, -9.6205) (-13.7585, -9.6156) knots 0 0 0 0 0.008307 0.018945 0.018945 0.018945 0.018945
  line L18 (-13.7585, -9.6156) -> (-13.6965, -9.9952)
  spline S27 degree 3 poles (-13.6965, -9.9952) (-13.7536, -10.0064) (-13.8609, -10.0273) (-13.9701, -10.0315) (-14.0211, -10.0334) knots 0 0 0 0 0.017427 0.032736 0.032736 0.032736 0.032736
  spline S28 degree 3 poles (-14.0211, -10.0334) (-14.0914, -10.0321) (-14.2173, -10.0297) (-14.333, -9.9809) (-14.384, -9.9594) knots 0 0 0 0 0.020853 0.037334 0.037334 0.037334 0.037334
  spline S29 degree 3 poles (-14.384, -9.9594) (-14.4235, -9.9335) (-14.4999, -9.8834) (-14.5441, -9.8035) (-14.5655, -9.7648) knots 0 0 0 0 0.013927 0.026964 0.026964 0.026964 0.026964
  spline S30 degree 3 poles (-14.5655, -9.7648) (-14.5806, -9.7027) (-14.621, -9.5365) (-14.6192, -9.3649) (-14.618, -9.2575) knots 0 0 0 0 0.019122 0.05117 0.05117 0.05117 0.05117
  line L19 (-14.618, -9.2575) -> (-14.618, -7.7988)
  line L20 (-14.618, -7.7988) -> (-14.9332, -7.7988)
  line L21 (-14.9332, -7.7988) -> (-14.9332, -7.4645)
  line L22 (-14.9332, -7.4645) -> (-14.618, -7.4645)
  line L23 (-14.618, -7.4645) -> (-14.618, -6.8366)
  line L24 (-14.618, -6.8366) -> (-14.1907, -6.5788)
  line L25 (-14.1907, -6.5788) -> (-14.1907, -7.4645)
  line L26 (-14.1907, -7.4645) -> (-13.7585, -7.4645)
  line L27 (-13.7585, -7.4645) -> (-13.7585, -7.7988)
  line L28 (-13.7585, -7.7988) -> (-14.1907, -7.7988)
  line L29 (-14.1907, -7.7988) -> (-14.1907, -9.2814)
  spline S31 degree 3 poles (-14.1907, -9.2814) (-14.1913, -9.332) (-14.1923, -9.4118) (-14.1745, -9.4894) (-14.168, -9.5177) knots 0 0 0 0 0.015111 0.023814 0.023814 0.023814 0.023814
  spline S32 degree 3 poles (-14.168, -9.5177) (-14.1591, -9.5344) (-14.1412, -9.5682) (-14.1098, -9.5902) (-14.094, -9.6013) knots 0 0 0 0 0.00558 0.011304 0.011304 0.011304 0.011304
  line L30 (-16.5853, -10) -> (-17.0341, -10)
  spline S33 degree 3 poles (-17.0341, -10) (-17.0545, -9.9522) (-17.0974, -9.852) (-17.1123, -9.7439) (-17.1201, -9.6872) knots 0 0 0 0 0.015508 0.032565 0.032565 0.032565 0.032565
  spline S34 degree 3 poles (-17.1201, -9.6872) (-17.1958, -9.7487) (-17.3372, -9.8634) (-17.5028, -9.9388) (-17.5796, -9.9737) knots 0 0 0 0 0.029128 0.054352 0.054352 0.054352 0.054352
  spline S35 degree 3 poles (-17.5796, -9.9737) (-17.6553, -9.9981) (-17.8094, -10.0477) (-17.9712, -10.0541) (-18.0535, -10.0573) knots 0 0 0 0 0.023732 0.048322 0.048322 0.048322 0.048322
  spline S36 degree 3 poles (-18.0535, -10.0573) (-18.1807, -10.0522) (-18.4145, -10.0429) (-18.6077, -9.9126) (-18.6958, -9.8532) knots 0 0 0 0 0.037297 0.068576 0.068576 0.068576 0.068576
  spline S37 degree 3 poles (-18.6958, -9.8532) (-18.7612, -9.7797) (-18.8939, -9.6309) (-18.9113, -9.4322) (-18.9202, -9.3315) knots 0 0 0 0 0.028701 0.058158 0.058158 0.058158 0.058158
  spline S38 degree 3 poles (-18.9202, -9.3315) (-18.9169, -9.2712) (-18.9104, -9.1523) (-18.8602, -9.0444) (-18.8354, -8.9913) knots 0 0 0 0 0.017942 0.035349 0.035349 0.035349 0.035349
  spline S39 degree 3 poles (-18.8354, -8.9913) (-18.8054, -8.9428) (-18.7461, -8.8471) (-18.6572, -8.7782) (-18.6134, -8.7442) knots 0 0 0 0 0.016982 0.033459 0.033459 0.033459 0.033459
  spline S40 degree 3 poles (-18.6134, -8.7442) (-18.5657, -8.7149) (-18.4685, -8.6552) (-18.3596, -8.6209) (-18.3042, -8.6033) knots 0 0 0 0 0.016728 0.034089 0.034089 0.034089 0.034089
  spline S41 degree 3 poles (-18.3042, -8.6033) (-18.2514, -8.5917) (-18.1252, -8.5639) (-17.9969, -8.5481) (-17.9222, -8.5389) knots 0 0 0 0 0.016212 0.038758 0.038758 0.038758 0.038758
  spline S42 degree 3 poles (-17.9222, -8.5389) (-17.7708, -8.5205) (-17.5117, -8.4892) (-17.2603, -8.4197) (-17.1559, -8.3909) knots 0 0 0 0 0.045692 0.078147 0.078147 0.078147 0.078147
  spline S43 degree 3 poles (-17.1559, -8.3909) (-17.1552, -8.3668) (-17.1541, -8.3294) (-17.1537, -8.292) (-17.1535, -8.2786) knots 0 0 0 0 0.007224 0.011224 0.011224 0.011224 0.011224
  spline S44 degree 3 poles (-17.1535, -8.2786) (-17.1552, -8.201) (-17.1582, -8.0641) (-17.2399, -7.9556) (-17.2752, -7.9086) knots 0 0 0 0 0.022588 0.039829 0.039829 0.039829 0.039829
  spline S45 degree 3 poles (-17.2752, -7.9086) (-17.3416, -7.8662) (-17.49, -7.7715) (-17.6669, -7.766) (-17.7647, -7.763) knots 0 0 0 0 0.023204 0.051906 0.051906 0.051906 0.051906
  spline S46 degree 3 poles (-17.7647, -7.763) (-17.8544, -7.7644) (-18.0122, -7.7668) (-18.152, -7.8384) (-18.2123, -7.8692) knots 0 0 0 0 0.026485 0.046548 0.046548 0.046548 0.046548
  spline S47 degree 3 poles (-18.2123, -7.8692) (-18.2583, -7.9158) (-18.3627, -8.0214) (-18.4033, -8.165) (-18.426, -8.2452) knots 0 0 0 0 0.019347 0.043872 0.043872 0.043872 0.043872
  line L31 (-18.426, -8.2452) -> (-18.8462, -8.1879)
  spline S48 degree 3 poles (-18.8462, -8.1879) (-18.8257, -8.1045) (-18.7873, -7.9485) (-18.6988, -7.8146) (-18.6576, -7.7522) knots 0 0 0 0 0.025533 0.047792 0.047792 0.047792 0.047792
  spline S49 degree 3 poles (-18.6576, -7.7522) (-18.6067, -7.6993) (-18.4988, -7.587) (-18.3544, -7.528) (-18.278, -7.4968) knots 0 0 0 0 0.021757 0.046207 0.046207 0.046207 0.046207
  spline S50 degree 3 poles (-18.278, -7.4968) (-18.1892, -7.4707) (-18.0015, -7.4155) (-17.8058, -7.4101) (-17.7026, -7.4072) knots 0 0 0 0 0.027628 0.058447 0.058447 0.058447 0.058447
  spline S51 degree 3 poles (-17.7026, -7.4072) (-17.6038, -7.4089) (-17.4245, -7.4119) (-17.2523, -7.4614) (-17.175, -7.4836) knots 0 0 0 0 0.029487 0.053518 0.053518 0.053518 0.053518
  spline S52 degree 3 poles (-17.175, -7.4836) (-17.1137, -7.5085) (-17.0019, -7.554) (-16.9156, -7.6379) (-16.8765, -7.6758) knots 0 0 0 0 0.019606 0.035791 0.035791 0.035791 0.035791
  spline S53 degree 3 poles (-16.8765, -7.6758) (-16.8468, -7.7183) (-16.7844, -7.8074) (-16.7571, -7.913) (-16.7428, -7.9683) knots 0 0 0 0 0.015412 0.03239 0.03239 0.03239 0.03239
  spline S54 degree 3 poles (-16.7428, -7.9683) (-16.7366, -8.0196) (-16.7207, -8.1511) (-16.7211, -8.2837) (-16.7214, -8.3646) knots 0 0 0 0 0.015483 0.039722 0.039722 0.039722 0.039722
  line L32 (-16.7214, -8.3646) -> (-16.7214, -8.9376)
  spline S55 degree 3 poles (-16.7214, -8.9376) (-16.7223, -9.1008) (-16.7239, -9.3539) (-16.7018, -9.606) (-16.6939, -9.6956) knots 0 0 0 0 0.048918 0.075885 0.075885 0.075885 0.075885
  spline S56 degree 3 poles (-16.6939, -9.6956) (-16.6824, -9.7482) (-16.6592, -9.8543) (-16.61, -9.9511) (-16.5853, -10) knots 0 0 0 0 0.016077 0.032437 0.032437 0.032437 0.032437
  circle A0 centre (-12.75, -15.2374) radius 2.7264
  spline S57 degree 3 poles (-12.2711, -9.704) (-12.1963, -9.6995) (-12.0515, -9.691) (-11.9275, -9.616) (-11.8677, -9.5798) knots 0 0 0 0 0.022124 0.042784 0.042784 0.042784 0.042784
  spline S58 degree 3 poles (-11.8677, -9.5798) (-11.8137, -9.5289) (-11.6955, -9.4173) (-11.6353, -9.2658) (-11.6027, -9.1835) knots 0 0 0 0 0.022003 0.048189 0.048189 0.048189 0.048189
  line L33 (-11.6027, -9.1835) -> (-11.1586, -9.2384)
  spline S59 degree 3 poles (-11.1586, -9.2384) (-11.1994, -9.3596) (-11.2783, -9.594) (-11.46, -9.7615) (-11.5477, -9.8424) knots 0 0 0 0 0.037666 0.07289 0.07289 0.07289 0.07289
  spline S60 degree 3 poles (-11.4666, -7.7534) (-11.3727, -7.8877) (-11.1691, -8.1789) (-11.153, -8.5354) (-11.1443, -8.7275) knots 0 0 0 0 0.048166 0.104492 0.104492 0.104492 0.104492
  spline S61 degree 3 poles (-11.1443, -8.7275) (-11.1444, -8.7434) (-11.1448, -8.7816) (-11.146, -8.8198) (-11.1467, -8.8421) knots 0 0 0 0 0.004775 0.011463 0.011463 0.011463 0.011463
  line L34 (-11.1467, -8.8421) -> (-13.0375, -8.8421)
  spline S62 degree 3 poles (-13.0375, -8.8421) (-13.0251, -8.9694) (-13.0022, -9.2043) (-12.8643, -9.3947) (-12.8012, -9.4819) knots 0 0 0 0 0.037564 0.069307 0.069307 0.069307 0.069307
  spline S63 degree 3 poles (-12.8012, -9.4819) (-12.7255, -9.5467) (-12.5727, -9.6774) (-12.3723, -9.6951) (-12.2711, -9.704) knots 0 0 0 0 0.029108 0.058759 0.058759 0.058759 0.058759
  line L35 (-10.1941, -8.6726) -> (-10.1941, -10)
  line L36 (-10.1941, -10) -> (-10.6238, -10)
  line L37 (-10.6238, -10) -> (-10.6238, -7.4645)
  line L38 (-10.6238, -7.4645) -> (-10.237, -7.4645)
  line L39 (-10.237, -7.4645) -> (-10.237, -7.8489)
  spline S64 degree 3 poles (-10.237, -7.8489) (-10.194, -7.7708) (-10.1207, -7.638) (-10.0095, -7.5354) (-9.9637, -7.4932) knots 0 0 0 0 0.026526 0.045117 0.045117 0.045117 0.045117
  spline S65 degree 3 poles (-9.9637, -7.4932) (-9.9209, -7.4681) (-9.8356, -7.4181) (-9.7371, -7.4109) (-9.6879, -7.4072) knots 0 0 0 0 0.014655 0.029228 0.029228 0.029228 0.029228
  spline S66 degree 3 poles (-9.6879, -7.4072) (-9.6135, -7.4141) (-9.4566, -7.4286) (-9.3187, -7.5053) (-9.2462, -7.5457) knots 0 0 0 0 0.022177 0.046743 0.046743 0.046743 0.046743
  line L40 (-9.2462, -7.5457) -> (-9.3943, -7.9444)
  spline S67 degree 3 poles (-9.3943, -7.9444) (-9.4457, -7.9173) (-9.5446, -7.865) (-9.6559, -7.8558) (-9.7094, -7.8513) knots 0 0 0 0 0.017235 0.033164 0.033164 0.033164 0.033164
  spline S68 degree 3 poles (-9.7094, -7.8513) (-9.7552, -7.8548) (-9.8466, -7.8619) (-9.9239, -7.9113) (-9.9625, -7.9361) knots 0 0 0 0 0.013537 0.027061 0.027061 0.027061 0.027061
  spline S69 degree 3 poles (-9.9625, -7.9361) (-9.9974, -7.9678) (-10.0695, -8.0332) (-10.1045, -8.1243) (-10.1224, -8.1712) knots 0 0 0 0 0.013953 0.028797 0.028797 0.028797 0.028797
  spline S70 degree 3 poles (-10.1224, -8.1712) (-10.1433, -8.2508) (-10.1865, -8.4151) (-10.1915, -8.5849) (-10.1941, -8.6726) knots 0 0 0 0 0.024588 0.050792 0.050792 0.050792 0.050792
  line L41 (-8.5587, -7.4645) -> (-8.5587, -10)
  line L42 (-8.5587, -10) -> (-8.9884, -10)
  line L43 (-8.9884, -10) -> (-8.9884, -7.4645)
  line L44 (-8.9884, -7.4645) -> (-8.5587, -7.4645)
  spline S71 degree 3 poles (-6.8373, -9.704) (-6.7624, -9.6995) (-6.6176, -9.691) (-6.4937, -9.616) (-6.4338, -9.5798) knots 0 0 0 0 0.022124 0.042784 0.042784 0.042784 0.042784
  spline S72 degree 3 poles (-6.4338, -9.5798) (-6.3799, -9.5289) (-6.2617, -9.4173) (-6.2015, -9.2658) (-6.1688, -9.1835) knots 0 0 0 0 0.022003 0.048189 0.048189 0.048189 0.048189
  line L45 (-6.1688, -9.1835) -> (-5.7248, -9.2384)
  spline S73 degree 3 poles (-5.7248, -9.2384) (-5.7656, -9.3596) (-5.8445, -9.594) (-6.0261, -9.7615) (-6.1139, -9.8424) knots 0 0 0 0 0.037666 0.07289 0.07289 0.07289 0.07289
  spline S74 degree 3 poles (-6.1139, -9.8424) (-6.219, -9.905) (-6.4422, -10.038) (-6.7022, -10.0506) (-6.8397, -10.0573) knots 0 0 0 0 0.036142 0.076727 0.076727 0.076727 0.076727
  spline S75 degree 3 poles (-6.8397, -10.0573) (-7.0128, -10.0458) (-7.3437, -10.0239) (-7.5997, -9.8146) (-7.7219, -9.7147) knots 0 0 0 0 0.050598 0.096759 0.096759 0.096759 0.096759
  spline S76 degree 3 poles (-7.7219, -9.7147) (-7.8168, -9.5823) (-8.0218, -9.2963) (-8.0387, -8.9433) (-8.0478, -8.7538) knots 0 0 0 0 0.047864 0.103406 0.103406 0.103406 0.103406
  spline S77 degree 3 poles (-8.0478, -8.7538) (-8.0388, -8.5579) (-8.0222, -8.1943) (-7.8142, -7.8975) (-7.7183, -7.7606) knots 0 0 0 0 0.057415 0.106574 0.106574 0.106574 0.106574
  spline S78 degree 3 poles (-7.7183, -7.7606) (-7.5983, -7.6575) (-7.3526, -7.4464) (-7.0291, -7.4205) (-6.8636, -7.4072) knots 0 0 0 0 0.046198 0.09464 0.09464 0.09464 0.09464
  spline S79 degree 3 poles (-6.8636, -7.4072) (-6.703, -7.4204) (-6.3883, -7.4463) (-6.1496, -7.6525) (-6.0327, -7.7534) knots 0 0 0 0 0.047001 0.092108 0.092108 0.092108 0.092108
  spline S80 degree 3 poles (-6.0327, -7.7534) (-5.9389, -7.8877) (-5.7353, -8.1789) (-5.7191, -8.5354) (-5.7104, -8.7275) knots 0 0 0 0 0.048166 0.104492 0.104492 0.104492 0.104492
  spline S81 degree 3 poles (-5.7104, -8.7275) (-5.7106, -8.7434) (-5.711, -8.7816) (-5.7121, -8.8198) (-5.7128, -8.8421) knots 0 0 0 0 0.004775 0.011463 0.011463 0.011463 0.011463
  line L46 (-5.7128, -8.8421) -> (-7.6037, -8.8421)
  spline S82 degree 3 poles (-7.6037, -8.8421) (-7.5913, -8.9694) (-7.5684, -9.2043) (-7.4305, -9.3947) (-7.3673, -9.4819) knots 0 0 0 0 0.037564 0.069307 0.069307 0.069307 0.069307
  spline S83 degree 3 poles (-7.3673, -9.4819) (-7.2916, -9.5467) (-7.1389, -9.6774) (-6.9384, -9.6951) (-6.8373, -9.704) knots 0 0 0 0 0.029108 0.058759 0.058759 0.058759 0.058759
  line L47 (-8.5587, -6.5) -> (-8.5587, -6.9942)
  line L48 (-8.5587, -6.9942) -> (-8.9884, -6.9942)
  line L49 (-8.9884, -6.9942) -> (-8.9884, -6.5)
  line L50 (-8.9884, -6.5) -> (-8.5587, -6.5)
  spline S84 degree 3 poles (-4.2732, -10.0573) (-4.4221, -10.0531) (-4.691, -10.0455) (-4.9229, -9.9117) (-5.0264, -9.852) knots 0 0 0 0 0.043843 0.07916 0.07916 0.07916 0.07916
  spline S85 degree 3 poles (-5.0264, -9.852) (-5.1055, -9.7717) (-5.2737, -9.6011) (-5.3282, -9.3671) (-5.3571, -9.2432) knots 0 0 0 0 0.033163 0.070487 0.070487 0.070487 0.070487
  line L51 (-5.3571, -9.2432) -> (-4.9321, -9.1763)
  spline S86 degree 3 poles (-4.9321, -9.1763) (-4.9164, -9.2551) (-4.8867, -9.4048) (-4.7822, -9.5155) (-4.7328, -9.5679) knots 0 0 0 0 0.023556 0.044735 0.044735 0.044735 0.044735
  spline S87 degree 3 poles (-4.7328, -9.5679) (-4.6692, -9.6075) (-4.5298, -9.6943) (-4.3651, -9.7006) (-4.2756, -9.704) knots 0 0 0 0 0.022104 0.048438 0.048438 0.048438 0.048438
  spline S88 degree 3 poles (-4.2756, -9.704) (-4.1872, -9.7019) (-4.0299, -9.6983) (-3.8953, -9.6184) (-3.8363, -9.5834) knots 0 0 0 0 0.02596 0.046233 0.046233 0.046233 0.046233
  spline S89 degree 3 poles (-3.8363, -9.5834) (-3.7945, -9.5427) (-3.7143, -9.4644) (-3.6999, -9.3536) (-3.693, -9.3005) knots 0 0 0 0 0.016943 0.032549 0.032549 0.032549 0.032549
  spline S90 degree 3 poles (-3.693, -9.3005) (-3.6986, -9.2544) (-3.7098, -9.161) (-3.7827, -9.1014) (-3.8196, -9.0713) knots 0 0 0 0 0.013391 0.02711 0.02711 0.02711 0.02711
  spline S91 degree 3 poles (-3.8196, -9.0713) (-3.8705, -9.0484) (-4.0117, -8.985) (-4.1625, -8.9488) (-4.2589, -8.9256) knots 0 0 0 0 0.016717 0.046363 0.046363 0.046363 0.046363
  spline S92 degree 3 poles (-4.2589, -8.9256) (-4.3934, -8.892) (-4.6161, -8.8362) (-4.8296, -8.7523) (-4.9142, -8.7191) knots 0 0 0 0 0.041539 0.068773 0.068773 0.068773 0.068773
  spline S93 degree 3 poles (-4.9142, -8.7191) (-4.9709, -8.6881) (-5.081, -8.6279) (-5.1552, -8.527) (-5.1912, -8.478) knots 0 0 0 0 0.019122 0.037119 0.037119 0.037119 0.037119
  spline S94 degree 3 poles (-5.1912, -8.478) (-5.2187, -8.4251) (-5.2741, -8.3184) (-5.2817, -8.1983) (-5.2855, -8.1378) knots 0 0 0 0 0.017681 0.035653 0.035653 0.035653 0.035653
  spline S95 degree 3 poles (-5.2855, -8.1378) (-5.2824, -8.0825) (-5.2762, -7.973) (-5.2305, -7.8733) (-5.2079, -7.8238) knots 0 0 0 0 0.016439 0.032594 0.032594 0.032594 0.032594
  spline S96 degree 3 poles (-5.2079, -7.8238) (-5.1797, -7.7777) (-5.1232, -7.6854) (-5.0388, -7.6178) (-4.9966, -7.5839) knots 0 0 0 0 0.016085 0.032187 0.032187 0.032187 0.032187
  spline S97 degree 3 poles (-4.9966, -7.5839) (-4.9578, -7.5595) (-4.8723, -7.5057) (-4.7759, -7.4752) (-4.7232, -7.4586) knots 0 0 0 0 0.013677 0.030182 0.030182 0.030182 0.030182
  spline S98 degree 3 poles (-4.7232, -7.4586) (-4.6637, -7.4436) (-4.5419, -7.4129) (-4.4163, -7.4092) (-4.352, -7.4072) knots 0 0 0 0 0.018344 0.037576 0.037576 0.037576 0.037576
  spline S99 degree 3 poles (-4.352, -7.4072) (-4.2578, -7.41) (-4.0792, -7.4152) (-3.9086, -7.4681) (-3.8279, -7.4932) knots 0 0 0 0 0.028105 0.053325 0.053325 0.053325 0.053325
  spline S100 degree 3 poles (-3.8279, -7.4932) (-3.7593, -7.5223) (-3.6315, -7.5764) (-3.5381, -7.6787) (-3.4949, -7.726) knots 0 0 0 0 0.022063 0.041059 0.041059 0.041059 0.041059
  spline S101 degree 3 poles (-3.4949, -7.726) (-3.4614, -7.7819) (-3.3886, -7.9037) (-3.3615, -8.0432) (-3.3469, -8.1187) knots 0 0 0 0 0.01941 0.042254 0.042254 0.042254 0.042254
  line L52 (-3.3469, -8.1187) -> (-3.7671, -8.176)
  spline S102 degree 3 poles (-3.7671, -8.176) (-3.7803, -8.115) (-3.8061, -7.9968) (-3.8916, -7.9116) (-3.933, -7.8704) knots 0 0 0 0 0.0183 0.035437 0.035437 0.035437 0.035437
  spline S103 degree 3 poles (-3.933, -7.8704) (-3.9868, -7.8384) (-4.1059, -7.7678) (-4.2448, -7.7631) (-4.3209, -7.7606) knots 0 0 0 0 0.018498 0.0409 0.0409 0.0409 0.0409
  spline S104 degree 3 poles (-4.3209, -7.7606) (-4.4074, -7.7613) (-4.5564, -7.7625) (-4.6882, -7.8301) (-4.7435, -7.8585) knots 0 0 0 0 0.025484 0.043902 0.043902 0.043902 0.043902
  spline S105 degree 3 poles (-4.7435, -7.8585) (-4.7804, -7.8911) (-4.8501, -7.9528) (-4.8637, -8.0444) (-4.8701, -8.0877) knots 0 0 0 0 0.014246 0.026941 0.026941 0.026941 0.026941